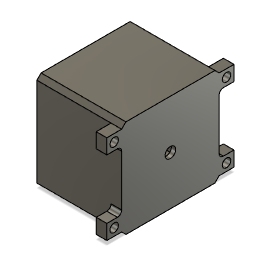
Крепление под шаговый v5 (Autodesk Fusion 360 design; units mm, degrees)
Autodesk Fusion 360 part; units mm, degrees
note: some values were not read from the file. Set by a fixed rule: which sketch regions a step uses.
sketch "Sketch1" plane through (0, 0, 0) normal (1, 0, 0) x (0, 0, -1)
  line L0 (0, 0) -> (-46, 0)
  line L1 (-46, 0) -> (-46, 46)
  line L2 (-46, 46) -> (0, 46)
  line L3 (0, 46) -> (0, 0)
  line L4 (-5.6171, 5.6171) -> (-5.4898, 5.6171)
  circle A0 centre (-23, 23) radius 2.5
  line L5 (0, 0) -> (-46, 46)
  line L6 (0, 46) -> (-46, 0)
  arc A1 (-37.1208, 37.5837) -> (-37.2298, 37.2298) centre (-35.7422, 36.9654) ccw
  line L7 (-7.5, 38.5) -> (-38.5, 38.5)
  line L8 (-38.5, 38.5) -> (-38.5, 7.5)
  line L9 (-38.5, 7.5) -> (-7.5, 7.5)
  line L10 (-7.5, 7.5) -> (-7.5, 38.5)
  line L11 (-7.5, 38.5) -> (-38.5, 7.5) construction
  line L12 (-38.5, 38.5) -> (-7.5, 7.5) construction
  circle A2 centre (-7.5, 38.5) radius 0.5
  circle A3 centre (-38.5, 38.5) radius 0.5
  circle A4 centre (-38.5, 7.5) radius 0.5
  circle A5 centre (-7.5, 7.5) radius 0.5
  point P0 (-23, 23)
  point P1 (-23, 23)
  point P2 (-23, 23)
  dimension "d1" = 46
  dimension "d9" = 5
  dimension "d50" = 46
  dimension "d51" = 31
  dimension "d52" = 31
  dimension "d53" = 1
  dimension "d54" = 1
  dimension "d55" = 1
  dimension "d56" = 1
  constraint horizontal L0
  constraint vertical L1
  constraint horizontal L2
  constraint vertical L3
  constraint coincident L0.start L3.end
  constraint coincident P2 P1
  constraint midpoint L5 P2
  constraint coincident L5 A1.end
  constraint coincident L5 L4.start
  constraint horizontal L7
  constraint perpendicular L7 L8
  constraint parallel L7 L9
  constraint parallel L8 L10
  constraint coincident L11 P2
  constraint coincident L12 P2
  constraint coincident L7.start L10.end
  constraint coincident L7.end L8.start
  constraint coincident L8.end L9.start
  constraint coincident L9.end L10.start
  measures "d1" distance of L0.start L0.end
  measures "d9" diameter of A0
  measures "d50" distance of L0.start L2.end
  measures "d51" distance of L8.end L9.end
  measures "d52" distance of L7.end L8.end
  measures "d53" diameter of A2
  measures "d54" diameter of A3
  measures "d55" diameter of A4
  measures "d56" diameter of A5
extrude "Extrude1" add sketch "Sketch1" along normal blind 34 contours L3 L5 L6 L10 A2 A5 | L0 L5 L6 L9 A4 A5 | L1 L5 L6 L8 A3 A4 | L2 L5 L6 L7 A2 A3 | L6 L8 A4 | L6 L9 A4 | L6 L10 A2 | L6 L7 A2 | L5 L9 A5 | L5 L10 A5 | L5 L7 A3 | L5 L8 A3 | L6 L8 A4 | L6 L9 A4 | A0 L5 L6 L8 A3 A4 | A0 L5 L6 L9 A4 A5 | L6 L10 A2 | L6 L7 A2 | A0 L5 L6 L7 A2 A3 | L5 L9 A5 | L5 L10 A5 | L5 L7 A3 | L5 L8 A3 | A0 L5 L6 L10 A2 A5
shell "Shell2" thickness 2 removed faces 1 at (0, 22.9406, 39.1645)
extrude "Extrude7" cut 1 faces at (0, 25.459, 25.9286) along direction (1, 0, 0) blind 32
extrude "Extrude8" add 1 faces at (0, 30, 45.3333) along direction (-1, 0, 0) blind 2
sketch "Sketch6" plane through (32, 0, 0) normal (-1, 0, 0) x (0, 0, 1)
  circle A0 centre (23, 23) radius 2.5
  line L0 (44, 44) -> (2, 44)
  line L1 (2, 44) -> (2, 2)
  line L2 (2, 2) -> (44, 2)
  line L3 (44, 2) -> (44, 44)
  circle A1 centre (23, 23) radius 11
  dimension "d62" = 22
  constraint concentric A0 A1
  measures "d62" diameter of A1
extrude "Extrude9" add 1 faces at (34, 6.8357, 23.0623) along direction (1, 0, 0) blind 2
extrude "Extrude10" cut sketch "Sketch6" against normal blind 2 contours A1
chamfer "Chamfer3" distance 2 angle 45 4 edges at (17, 46, 46) (17, 46, 0) (17, 0, 0) (17, 0, 46)
sketch "Sketch7" plane through (0, 0, 0) normal (0, -1, 0) x (1, 0, 0)
  line L0 (36, 44) -> (-2, 44)
  line L1 (-2, 44) -> (-2, 2)
  line L2 (-2, 2) -> (36, 2)
  line L3 (36, 2) -> (36, 44)
  line L4 (-2, 0) -> (-2, 18.65)
  line L5 (-2, 18.65) -> (1, 18.65)
  line L6 (1, 18.65) -> (6, 18.65)
  line L7 (6, 18.65) -> (6, 26.65)
  line L8 (6, 26.65) -> (1, 26.65)
  line L9 (1, 26.65) -> (1, 18.65)
  dimension "d68" = 18.65
  dimension "d69" = 3
  dimension "d70" = 5
  dimension "d71" = 8
  constraint parallel L1 L4
  constraint perpendicular L4 L5
  constraint horizontal L6
  constraint vertical L7
  constraint horizontal L8
  constraint vertical L9
  measures "d68" distance of L4.start L4.end
  measures "d69" distance of L4.end L5.end
  measures "d70" distance of L5.end L6.end
  measures "d71" distance of L5.end L8.end
extrude "Extrude11" cut sketch "Sketch7" against normal blind 5 contours L6 L7 L8 L9
sketch "Sketch8" plane through (36, 0, 0) normal (1, 0, 0) x (0, 0, -1)
  circle A0 centre (-23, 23) radius 2.5
  line L0 (-46, 2) -> (-44, 0)
  line L1 (-44, 0) -> (-2, 0)
  line L2 (-2, 0) -> (0, 2)
  line L3 (0, 2) -> (0, 44)
  line L4 (0, 44) -> (-2, 46)
  line L5 (-2, 46) -> (-44, 46)
  line L6 (-44, 46) -> (-46, 44)
  line L7 (-46, 44) -> (-46, 2)
  line L8 (-46, 44) -> (-53, 44)
  line L9 (-53, 44) -> (-53, 37)
  line L10 (-53, 37) -> (-46, 37)
  line L11 (-46, 37) -> (-46, 44)
  line L12 (0, 44) -> (7, 44)
  line L13 (7, 44) -> (7, 37)
  line L14 (7, 37) -> (0, 37)
  line L15 (0, 37) -> (0, 44)
  line L16 (0, 2) -> (7, 2)
  line L17 (7, 2) -> (7, 9)
  line L18 (7, 9) -> (0, 9)
  line L19 (0, 9) -> (0, 2)
  line L20 (-46, 2) -> (-53, 2)
  line L21 (-53, 2) -> (-53, 9)
  line L22 (-53, 9) -> (-46, 9)
  line L23 (-46, 9) -> (-46, 2)
  line L24 (-46, 44) -> (-53, 37)
  line L25 (-53, 44) -> (-46, 37)
  line L26 (-53, 9) -> (-53, 8.7308)
  line L27 (-46, 2) -> (-53, 9)
  line L28 (-53, 2) -> (-46, 9)
  line L29 (0, 2) -> (7, 9)
  line L30 (0, 9) -> (7, 2)
  line L31 (0, 37) -> (7, 44)
  line L32 (0, 44) -> (7, 37)
  circle A1 centre (3.5, 40.5) radius 2
  circle A2 centre (3.5, 5.5) radius 2
  circle A3 centre (-49.5, 5.5) radius 2
  circle A4 centre (-49.5, 40.5) radius 2
  dimension "d74" = 7
  dimension "d75" = 7
  dimension "d76" = 7
  dimension "d77" = 7
  dimension "d78" = 7
  dimension "d79" = 7
  dimension "d80" = 7
  dimension "d81" = 7
  dimension "d82" = 4
  dimension "d83" = 4
  dimension "d84" = 4
  dimension "d85" = 4
  constraint horizontal L8
  constraint vertical L9
  constraint horizontal L10
  constraint vertical L11
  constraint coincident L6.end L7.start
  constraint horizontal L12
  constraint vertical L13
  constraint horizontal L14
  constraint vertical L15
  constraint coincident L3.end L4.start
  constraint horizontal L16
  constraint vertical L17
  constraint horizontal L18
  constraint vertical L19
  constraint coincident L2.end L3.start
  constraint horizontal L20
  constraint vertical L21
  constraint horizontal L22
  constraint vertical L23
  constraint coincident L0.start L7.end
  constraint coincident L21 L26.end
  constraint midpoint L31 A1.centre
  constraint midpoint L29 A2.centre
  constraint midpoint L27 A3.centre
  constraint midpoint L24 A4.centre
  measures "d74" distance of L6.end L8.end
  measures "d75" distance of L6.end L10.end
  measures "d76" distance of L3.end L12.end
  measures "d77" distance of L3.end L14.end
  measures "d78" distance of L2.end L16.end
  measures "d79" distance of L2.end L18.end
  measures "d80" distance of L0.start L20.end
  measures "d81" distance of L0.start L22.end
  measures "d82" diameter of A1
  measures "d83" diameter of A2
  measures "d84" diameter of A3
  measures "d85" diameter of A4
extrude "Extrude12" add sketch "Sketch8" against normal blind 5 contours L7 L23 L27 L28 A3 | L20 L27 L28 A3 | L22 L27 L28 A3 | L21 L26 L27 L28 A3 | L7 L11 L24 L25 A4 | L10 L24 L25 A4 | L16 L29 L30 A2 | L3 L19 L29 L30 A2 | L8 L24 L25 A4 | L9 L24 L25 A4 | L18 L29 L30 A2 | L17 L29 L30 A2 | L14 L31 L32 A1 | L3 L15 L31 L32 A1 | L12 L31 L32 A1 | L13 L31 L32 A1
fillet "Fillet2" radius 2 4 edges at (33.5, 37, 46) (33.5, 9, 46) (33.5, 9, 0) (33.5, 37, 0)
extrude "Extrude13" add 1 faces at (-2, 1.3333, 30) along direction (-1, 0, 0) blind 2
extrude "Extrude2" [suppressed]
sketch "Sketch3" plane through (32, 0, 0) normal (-1, 0, 0) x (0, 0, 1)
  circle A0 centre (22, 22) radius 2.5
  circle A1 centre (22, 22) radius 12.5
  line L0 (44, 0) -> (44, 44)
  line L1 (44, 44) -> (0, 44)
  line L2 (0, 44) -> (0, 0)
  line L3 (0, 0) -> (44, 0)
  dimension "d16" = 25
  constraint concentric A0 A1
  measures "d16" diameter of A1
extrude "Extrude3" [suppressed]
sketch "Sketch4" plane through (34, 0, 0) normal (1, 0, 0) x (0, 0, -1)
  line L0 (-44, 0) -> (0, 0)
  line L1 (0, 0) -> (0, 44)
  line L2 (0, 44) -> (-44, 44)
  line L3 (-44, 44) -> (-44, 0)
  circle A0 centre (-22, 22) radius 2.5
  line L4 (-39.9874, 35) -> (-47.9874, 35)
  line L5 (-47.9874, 35) -> (-47.9874, 40)
  line L6 (-47.9874, 40) -> (-39.9874, 40)
  line L7 (-39.9874, 40) -> (-39.9874, 35)
  line L8 (-40, 4) -> (-48, 4)
  line L9 (-48, 4) -> (-48, 9)
  line L10 (-48, 9) -> (-40, 9)
  line L11 (-40, 9) -> (-40, 4)
  line L12 (-4, 4) -> (4, 4)
  line L13 (4, 4) -> (4, 9)
  line L14 (4, 9) -> (-4, 9)
  line L15 (-4, 9) -> (-4, 4)
  line L16 (-3.9874, 40) -> (4.0126, 40)
  line L17 (4.0126, 40) -> (4.0126, 35)
  line L18 (4.0126, 35) -> (-3.9874, 35)
  line L19 (-3.9874, 35) -> (-3.9874, 40)
  circle A1 centre (-44.9824, 36.5) radius 2
  circle A2 centre (-44.9824, 5.461) radius 2
  line L20 (-22, 22) -> (-22, 48)
  circle A3 centre (0.9824, 5.461) radius 2
  circle A4 centre (0.9824, 36.5) radius 2
  dimension "d22" = 8
  dimension "d23" = 8
  dimension "d24" = 5
  dimension "d25" = 8
  dimension "d26" = 5
  dimension "d27" = 8
  dimension "d28" = 5
  dimension "d29" = 5
  dimension "d30" = 36
  dimension "d31" = 26
  dimension "d32" = 17.9874
  dimension "d33" = 13
  dimension "d34" = 13
  dimension "d35" = 26
  dimension "d36" = 36
  dimension "d37" = 18
  dimension "d38" = 4
  dimension "d39" = 4
  constraint horizontal L4
  constraint vertical L5
  constraint horizontal L6
  constraint vertical L7
  constraint horizontal L8
  constraint vertical L9
  constraint horizontal L10
  constraint vertical L11
  constraint horizontal L12
  constraint vertical L13
  constraint horizontal L14
  constraint vertical L15
  constraint horizontal L16
  constraint vertical L17
  constraint horizontal L18
  constraint vertical L19
  constraint coincident A0.centre L20.start
  constraint perpendicular L2 L20
  constraint symmetric A1 L20 A4
  constraint symmetric A2 L20 A3
  measures "d22" distance of L4.start L4.end
  measures "d23" distance of L8.start L8.end
  measures "d24" distance of L8.start L10.end
  measures "d25" distance of L12.start L12.end
  measures "d26" distance of L12.start L14.end
  measures "d27" distance of L16.start L16.end
  measures "d28" distance of L16.start L18.end
  measures "d29" distance of L4 L6
  measures "d30" distance of L7 L19
  measures "d31" distance of L4 L10
  measures "d32" horizontal distance of A0.centre L4.start
  measures "d33" vertical distance of A0.centre L4.start
  measures "d34" distance of A0.centre L18
  measures "d35" distance of L14 L18
  measures "d36" distance of L11 L15
  measures "d37" distance of A0.centre L11
  measures "d38" diameter of A1
  measures "d39" diameter of A2
extrude "Extrude5" [suppressed]
sketch "Sketch5" plane through (0, 0, 0) normal (0, -1, 0) x (1, 0, 0)
  line L0 (34, 0) -> (34, 44)
  line L1 (-3, 0) -> (-3, 14)
  line L2 (-3, 14) -> (7, 14)
  line L3 (7, 14) -> (7, 30)
  line L4 (7, 30) -> (-3, 30)
  line L5 (-3, 30) -> (-3, 14)
  line L6 (29, 44) -> (29, 0)
  line L7 (29, 0) -> (34, 0)
  line L8 (34, 44) -> (29, 44)
  dimension "d45" = 14
  dimension "d46" = 10
  dimension "d47" = 16
  constraint horizontal L2
  constraint vertical L3
  constraint horizontal L4
  constraint vertical L5
  measures "d45" distance of L1.start L1.end
  measures "d46" distance of L1.end L2.end
  measures "d47" distance of L1.end L4.end
